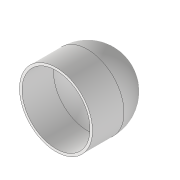
# Autodesk Inventor part: Behaelter_1
Saved by Autodesk Inventor 2020 (Build 240168000, 168)
## iProperties
Created: 2020-04-19
Part Number: Behaelter_1
Material: Generisch
Document SubType Name: Modeling
Designer: franz
Density: 1 g/cm^3
Appearance: Vorgabe
Author: franz
Autodesk Inventor part; units mm, degrees
ref_plane "YZ Plane" through (0, 0, 0) normal (1, 0, 0) x (0, 1, 0)
ref_plane "XZ Plane" through (0, 0, 0) normal (0, 1, 0) x (-1, 0, 0)
ref_plane "XY Plane" through (0, 0, 0) normal (0, 0, 1) x (1, 0, 0)
sketch "Skizze1" plane through (0, 0, 0) normal (0, 1, 0) x (-1, 0, 0)
  line L0 (0, 76.7155) -> (0, -97.245)
  line L1 (0, -132.0371) -> (0, 111.5076) projected
  line L2 (43, 0) -> (40, 0)
  line L3 (40, 0) -> (40, -37)
  arc A0 (0, -77) -> (40, -37) centre (0, -37) ccw
  arc A1 (0, -80) -> (43, -37) centre (0, -37) ccw
  line L4 (43, -37) -> (43, 0)
  line L5 (40, 0) -> (43, 0)
  line L6 (0, -77) -> (0, -45.7143)
  line L7 (62.2867, 0) -> (-10.3811, 0) projected
  point P0 (0, 0)
  dimension "d0" = 3
  dimension "d1" = 3
  dimension "d2" = 80
  dimension "d3" = 80
  constraints: 12 end point, 4 point on circle, 3 point on line, 2 centre point, 2 collinear, 2 perpendicular, 2 vertical, 1 coincident, 1 horizontal, 1 tangent
  measures "d0" distance between parallel lines of L3 L4
  measures "d1" distance of A1.start L6.start
  measures "d2" distance from line of A1.start L2
  measures "d3" diameter of L3 L0
revolve "Umdrehung1" add sketch "Skizze1" angle 360 about axis through (0, 0, 76.7155) along (0, 0, -1) contours A0 L3 L2 L4 A1 L0
equation "\"d1\" = d0"
